Autodesk Fusion 360 part; units mm, degrees
note: some values were not read from the file. Chosen so that the rebuilt part matches the saved one: which bodies a step acts on; which face or edge a step refers to. Set by a fixed rule: which sketch regions a step uses.
(part 2 of 2)
extrude "Extrude3''" [suppressed] in component "Cube HalfSpace"
fillet "Fillet1''" [suppressed] in component "Cube HalfSpace"
extrude "Extrude4''" [suppressed] in component "Cube HalfSpace"
extrude "Extrude5''" [suppressed] in component "Cube HalfSpace"
extrude "Extrude6''" [suppressed] in component "Cube HalfSpace"
extrude "Extrude7''" [suppressed] in component "Cube HalfSpace"
fillet "Fillet2''" [suppressed] in component "Cube HalfSpace"
sketch "Sketch6 (3)" plane through (0, -18.4, 0) normal (0, -1, 0) x (1, 0, 0) in component "Cube HalfSpace"
  arc A0 (45.1, 20) -> (45.1, 10) centre (45.1, 15) ccw
  line L0 (45.1, 10) -> (50.15, 10)
  line L1 (50.15, 10) -> (50.15, 20)
  line L2 (50.15, 20) -> (45.1, 20)
  circle A1 centre (45.1, 15) radius 2.5
  circle A2 centre (45.1, 15) radius 5.1 construction
  dimension "d54_1" = 8.3333
  dimension "d63_1" = 16.8667
  constraint concentric A0 A1
  constraint concentric A0 A2
ref_plane "WorkPlane1" through (45.125, -20.9, 15) normal (0, -1, 0) x (1, 0, 0) in component "Cube HalfSpace"
sketch "Sketch7 (3)" plane through (35.7, -20.9, 16.5) normal (0, -1, 0) x (1, 0, 0) in component "Cube HalfSpace"
  point P0 (9.4, -1.5)
loft "Loft1''" [suppressed] in component "Cube HalfSpace"
sketch "Sketch8" plane through (0, -6.6, 0) normal (0, 1, 0) x (-1, 0, 0) in component "Cube HalfSpace"
  arc A0 (-45.1, 10) -> (-45.1, 20) centre (-45.1, 15) ccw
  line L0 (-45.1, 20) -> (-50.15, 20)
  line L1 (-50.15, 20) -> (-50.15, 10)
  line L2 (-50.15, 10) -> (-45.1, 10)
  circle A1 centre (-45.1, 15) radius 2.5
  circle A2 centre (-45.1, 15) radius 2.5
  dimension "d64_1" = 8.3333
  constraint concentric A1 A2
ref_plane "WorkPlane2" through (45.125, -4.1, 15) normal (0, 1, 0) x (-1, 0, 0) in component "Cube HalfSpace"
sketch "Sketch9" plane through (35.7, -4.1, 16.5) normal (0, 1, 0) x (1, 0, 0) in component "Cube HalfSpace"
  point P0 (9.4, 1.5)
loft "Loft2" [suppressed] in component "Cube HalfSpace"
sketch "Sketch10 (3)" plane through (0, -18.5, 0) normal (0, 1, 0) x (-1, 0, 0) in component "Cube HalfSpace"
  line L0 (-46.6, 20) -> (-50.1, 16.5)
  line L1 (-50.1, 16.5) -> (-50.1, 9.9)
  line L2 (-50.1, 9.9) -> (-40, 9.9)
  line L3 (-40, 9.9) -> (-40, 20)
  line L4 (-40, 20) -> (-46.6, 20)
  circle A0 centre (-45.1, 15) radius 2.5
  circle A1 centre (-45.1, 15) radius 2.6
  dimension "d57_1" = 0.1
ref_plane "WorkPlane3" through (36.3, -18.1, 16.2) normal (0, 1, 0) x (-1, 0, 0) in component "Cube HalfSpace"
sketch "Sketch11 (3)" plane through (35.4, -18.1, 16.3) normal (0, 1, 0) x (1, 0, 0) in component "Cube HalfSpace"
  point P0 (0.95, 0.05)
loft "Loft3''" [suppressed] in component "Cube HalfSpace"
ref_plane "WorkPlane4" through (30.1, -10, 20) normal (0, 1, 0) x (-1, 0, 0) in component "Cube HalfSpace"
mirror "Mirror1" [suppressed] in component "Cube HalfSpace"
ref_plane "WorkPlane5" through (10, -10, 20) normal (1, 0, 0) x (0, 1, 0) in component "Cube HalfSpace"
sketch "Sketch12 (3)" plane through (4.1, 0, 0) normal (-1, 0, 0) x (0, -1, 0) in component "Cube HalfSpace"
  arc A0 (3.75, 12.5) -> (3.75, 20) centre (3.75, 16.25) ccw
  line L0 (3.75, 20) -> (-0.05, 20)
  line L1 (-0.05, 20) -> (-0.05, 12.5)
  line L2 (-0.05, 12.5) -> (3.75, 12.5)
  circle A1 centre (3.75, 16.25) radius 2
  dimension "d66_1" = 8.3333
  constraint concentric A0 A1
ref_plane "WorkPlane6" through (2.1, -3.725, 16.25) normal (-1, 0, 0) x (0, -1, 0) in component "Cube HalfSpace"
sketch "Sketch13 (3)" plane through (2.1, -3.55, 16.25) normal (-1, 0, 0) x (0, 1, 0) in component "Cube HalfSpace"
  point P0 (-0.2, 0)
loft "Loft4''" [suppressed] in component "Cube HalfSpace"
sketch "Sketch14 (3)" plane through (4, 0, 0) normal (1, 0, 0) x (0, 1, 0) in component "Cube HalfSpace"
  line L0 (0, 16.5) -> (-3.5, 20)
  line L1 (-3.5, 20) -> (-7.6, 20)
  line L2 (-7.6, 20) -> (-7.6, 12.4)
  line L3 (-7.6, 12.4) -> (0, 12.4)
  line L4 (0, 12.4) -> (0, 16.5)
  circle A0 centre (-3.75, 16.25) radius 2
  circle A1 centre (-3.75, 16.25) radius 2.1
  dimension "d68_1" = 0.1
ref_plane "WorkPlane7" through (2.1, -3.8, 16.2) normal (1, 0, 0) x (0, 1, 0) in component "Cube HalfSpace"
sketch "Sketch15 (3)" plane through (2.1, -3.85, 16.05) normal (1, 0, 0) x (0, 1, 0) in component "Cube HalfSpace"
  point P0 (0.1, 0.2)
loft "Loft5''" [suppressed] in component "Cube HalfSpace"
mirror "Mirror2''" [suppressed] in component "Cube HalfSpace"
sketch "Sketch16 (3)" plane through (0, -4.1, 0) normal (0, 1, 0) x (-1, 0, 0) in component "Cube HalfSpace"
  arc A0 (-23.85, 7.5) -> (-23.85, 0) centre (-23.85, 3.75) ccw
  line L0 (-23.85, 0) -> (-16.25, 0)
  arc A1 (-16.25, 0) -> (-16.25, 7.5) centre (-16.25, 3.75) ccw
  line L1 (-16.25, 7.5) -> (-23.85, 7.5)
  circle A2 centre (-23.85, 3.75) radius 2
  circle A3 centre (-16.25, 3.75) radius 2
  dimension "d72_1" = 8.3333
  dimension "d73_1" = 8.3333
  constraint concentric A0 A2
  constraint concentric A1 A3
ref_plane "WorkPlane8" through (20.05, -2.1, 3.75) normal (0, 1, 0) x (-1, 0, 0) in component "Cube HalfSpace"
sketch "Sketch17 (3)" plane through (20.2, -2.1, 3.75) normal (0, 1, 0) x (1, 0, 0) in component "Cube HalfSpace"
  point P0 (3.65, 0)
  point P1 (-3.95, 0)
loft "Loft6''" [suppressed] in component "Cube HalfSpace"
loft "Loft7''" [suppressed] in component "Cube HalfSpace"
sketch "Sketch18 (3)" plane through (0, -4, 0) normal (0, -1, 0) x (1, 0, 0) in component "Cube HalfSpace"
  line L0 (16.5, 0) -> (20, 3.5)
  line L1 (20, 3.5) -> (20, 7.6)
  line L2 (20, 7.6) -> (12.4, 7.6)
  line L3 (12.4, 7.6) -> (12.4, 0)
  line L4 (12.4, 0) -> (16.5, 0)
  circle A0 centre (16.25, 3.75) radius 2
  circle A1 centre (16.25, 3.75) radius 2.1
  dimension "d75_1" = 0.1
ref_plane "WorkPlane9" through (16.2, -1.9, 3.8) normal (0, -1, 0) x (1, 0, 0) in component "Cube HalfSpace"
sketch "Sketch19 (3)" plane through (16.15, -1.9, 3.95) normal (0, -1, 0) x (1, 0, 0) in component "Cube HalfSpace"
  point P0 (0.1, -0.2)
loft "Loft8''" [suppressed] in component "Cube HalfSpace"
sketch "Sketch20 (3)" plane through (0, -4, 0) normal (0, -1, 0) x (1, 0, 0) in component "Cube HalfSpace"
  line L0 (20.1, 3.5) -> (23.6, 0)
  line L1 (23.6, 0) -> (27.7, 0)
  line L2 (27.7, 0) -> (27.7, 7.6)
  line L3 (27.7, 7.6) -> (20.1, 7.6)
  line L4 (20.1, 7.6) -> (20.1, 3.5)
  circle A0 centre (23.85, 3.75) radius 2
  circle A1 centre (23.85, 3.75) radius 2.1
  point P0 (23.85, 3.75)
  dimension "d77_1" = 0.1
ref_plane "WorkPlane10" through (23.9, -1.9, 3.8) normal (0, -1, 0) x (1, 0, 0) in component "Cube HalfSpace"
sketch "Sketch21 (3)" plane through (24.25, -1.9, 3.95) normal (0, -1, 0) x (1, 0, 0) in component "Cube HalfSpace"
  point P0 (-0.4, -0.2)
loft "Loft9''" [suppressed] in component "Cube HalfSpace"
mirror "Mirror3''" [suppressed] in component "Cube HalfSpace"
mirror "Mirror4''" [suppressed] in component "Cube HalfSpace"
combine "Combine2''" [suppressed] in component "Cube HalfSpace"
mirror "Mirror5''" [suppressed] in component "Cube HalfSpace"
combine "Combine3''" [suppressed] in component "Cube HalfSpace"
combine "Combine4''" [suppressed] in component "Cube HalfSpace"
sketch "Sketch1 (4)" plane through (0, 0, 0) normal (0, 0, 1) x (1, 0, 0) in component "Cube Hinge"
  line L0 (0, 0) -> (20, 0)
  line L1 (20, 0) -> (20, -20)
  line L2 (20, -20) -> (0, -20)
  line L3 (0, -20) -> (0, 0)
  line L4 (20.2, 0) -> (40.2, 0)
  line L5 (40.2, 0) -> (40.2, -20)
  line L6 (40.2, -20) -> (20.2, -20)
  line L7 (20.2, -20) -> (20.2, 0)
  dimension "d1_2" = 50
  dimension "d2_2" = 50
  dimension "d3_2" = 50
  dimension "d4_2" = 50
  dimension "d5_2" = 0.2
  constraint horizontal L0
  constraint vertical L1
  constraint horizontal L2
  constraint vertical L3
  constraint coincident L0.start L3.end
  constraint horizontal L4
  constraint vertical L5
  constraint horizontal L6
  constraint vertical L7
  constraint collinear L0 L4
  measures "d5_2" distance of L1 L7
extrude "Extrude1'''" [suppressed] in component "Cube Hinge"
sketch "Sketch2 (4)" plane through (0, 0, 0) normal (0, 0, -1) x (1, 0, 0) in component "Cube Hinge"
  line L0 (20, 20) -> (0, 20)
  line L1 (0, 20) -> (0, 0)
  line L2 (0, 0) -> (20, 0)
  line L3 (20, 0) -> (20, 20)
  line L4 (20, 4) -> (12.4, 4)
  line L5 (12.4, 4) -> (12.4, 16)
  line L6 (12.4, 16) -> (20, 16)
  line L7 (20, 16) -> (20, 4)
  line L8 (20.1, 4.2) -> (12.6, 4.2)
  line L9 (12.6, 4.2) -> (12.6, 15.8)
  line L10 (12.6, 15.8) -> (20.1, 15.8)
  line L11 (20.1, 15.8) -> (20.1, 4.2)
  line L12 (0, 10) -> (20, 10) construction
  dimension "d8_2" = 0.1
  dimension "d9_2" = 0.2
  dimension "d10_2" = 0.2
  dimension "d11_2" = 0.2
  dimension "d12_2" = 25
  dimension "d13_2" = 16.7667
  constraint horizontal L4
  constraint vertical L5
  constraint horizontal L6
  constraint vertical L7
  constraint coincident L3 L4.start
  constraint horizontal L8
  constraint vertical L9
  constraint horizontal L10
  constraint vertical L11
  constraint midpoint L1 L12.start
  constraint midpoint L3 L12.end
  constraint symmetric L4 L6 L12
  measures "d8_2" distance of L7 L11
  measures "d9_2" distance of L4 L8
  measures "d10_2" distance of L6 L10
  measures "d11_2" distance of L5 L9
sketch "Sketch3 (4)" plane through (0, 0, 0) normal (0, 0, -1) x (1, 0, 0) in component "Cube Hinge"
  line L0 (40.2, 20) -> (20.2, 20)
  line L1 (20.2, 20) -> (20.2, 0)
  line L2 (20.2, 0) -> (40.2, 0)
  line L3 (40.2, 0) -> (40.2, 20)
  line L4 (40.2, 10) -> (20.2, 10) construction
  line L5 (27.8, 4) -> (20.2, 4)
  line L6 (20.2, 4) -> (20.2, 16)
  line L7 (20.2, 16) -> (27.8, 16)
  line L8 (27.8, 16) -> (27.8, 4)
  line L9 (27.6, 4.2) -> (20.1, 4.2)
  line L10 (20.1, 4.2) -> (20.1, 15.8)
  line L11 (20.1, 15.8) -> (27.6, 15.8)
  line L12 (27.6, 15.8) -> (27.6, 4.2)
  dimension "d19_2" = 0.2
  dimension "d20_2" = 0.2
  dimension "d21_2" = 0.2
  dimension "d22_2" = 25
  dimension "d23_2" = 0.1
  dimension "d24_2" = 16.7667
  constraint midpoint L3 L4.start
  constraint midpoint L1 L4.end
  constraint horizontal L5
  constraint vertical L6
  constraint horizontal L7
  constraint vertical L8
  constraint coincident L1 L6.end
  constraint horizontal L9
  constraint vertical L10
  constraint horizontal L11
  constraint vertical L12
  constraint symmetric L4 L5 L7
  measures "d19_2" distance of L5 L9
  measures "d20_2" distance of L8 L12
  measures "d21_2" distance of L7 L11
  measures "d23_2" distance of L6 L10
sketch "Sketch4 (4)" plane through (0, 0, 20) normal (0, 0, 1) x (-1, 0, 0) in component "Cube Hinge"
  line L0 (0, 20) -> (-20, 20)
  line L1 (-20, 20) -> (-20, 0)
  line L2 (-20, 0) -> (0, 0)
  line L3 (0, 0) -> (0, 20)
  line L4 (-10, 20) -> (-10, 0) construction
  line L5 (-16, 7.6) -> (-4, 7.6)
  line L6 (-4, 7.6) -> (-4, 0)
  line L7 (-4, 0) -> (-16, 0)
  line L8 (-16, 0) -> (-16, 7.6)
  line L9 (-15.8, 7.4) -> (-4.2, 7.4)
  line L10 (-4.2, 7.4) -> (-4.2, -0.1)
  line L11 (-4.2, -0.1) -> (-15.8, -0.1)
  line L12 (-15.8, -0.1) -> (-15.8, 7.4)
  dimension "d25_2" = 0.1
  dimension "d26_2" = 0.2
  dimension "d27_2" = 0.2
  dimension "d28_2" = 25
  dimension "d29_2" = 0.2
  dimension "d30_2" = 16.7667
  constraint midpoint L0 L4.start
  constraint midpoint L2 L4.end
  constraint horizontal L5
  constraint vertical L6
  constraint horizontal L7
  constraint vertical L8
  constraint coincident L2 L6.end
  constraint horizontal L9
  constraint vertical L10
  constraint horizontal L11
  constraint vertical L12
  constraint symmetric L4 L6 L8
  measures "d25_2" distance of L7 L11
  measures "d26_2" distance of L8 L12
  measures "d27_2" distance of L6 L10
  measures "d29_2" distance of L5 L9
sketch "Sketch5 (4)" plane through (0, 0, 20) normal (0, 0, 1) x (-1, 0, 0) in component "Cube Hinge"
  line L0 (-20.2, 20) -> (-40.2, 20)
  line L1 (-40.2, 20) -> (-40.2, 0)
  line L2 (-40.2, 0) -> (-20.2, 0)
  line L3 (-20.2, 0) -> (-20.2, 20)
  line L4 (-40.2, 10) -> (-20.2, 10) construction
  line L5 (-40.2, 16) -> (-32.6, 16)
  line L6 (-32.6, 16) -> (-32.6, 4)
  line L7 (-32.6, 4) -> (-40.2, 4)
  line L8 (-40.2, 4) -> (-40.2, 16)
  line L9 (-40.3, 15.8) -> (-32.8, 15.8)
  line L10 (-32.8, 15.8) -> (-32.8, 4.2)
  line L11 (-32.8, 4.2) -> (-40.3, 4.2)
  line L12 (-40.3, 4.2) -> (-40.3, 15.8)
  dimension "d31_2" = 0.1
  dimension "d32_2" = 0.2
  dimension "d33_2" = 0.2
  dimension "d34_2" = 0.2
  dimension "d35_2" = 16.7667
  dimension "d36_2" = 25
  constraint midpoint L1 L4.start
  constraint midpoint L3 L4.end
  constraint horizontal L5
  constraint vertical L6
  constraint horizontal L7
  constraint vertical L8
  constraint coincident L1 L5.start
  constraint horizontal L9
  constraint vertical L10
  constraint horizontal L11
  constraint vertical L12
  constraint symmetric L4 L5 L7
  measures "d31_2" distance of L8 L12
  measures "d32_2" distance of L7 L11
  measures "d33_2" distance of L5 L9
  measures "d34_2" distance of L6 L10
chamfer "Chamfer1'''" [suppressed] in component "Cube Hinge"
extrude "Extrude2'''" [suppressed] in component "Cube Hinge"
extrude "Extrude3'''" [suppressed] in component "Cube Hinge"
fillet "Fillet1'''" [suppressed] in component "Cube Hinge"
sketch "Sketch16 (4)" plane through (0, -4.2, 0) normal (0, 1, 0) x (-1, 0, 0) in component "Cube Hinge"
  arc A0 (-23.85, 7.5) -> (-23.85, 0) centre (-23.85, 3.75) ccw
  line L0 (-23.85, 0) -> (-16.35, 0)
  arc A1 (-16.35, 0) -> (-16.35, 7.5) centre (-16.35, 3.75) ccw
  line L1 (-16.35, 7.5) -> (-23.85, 7.5)
  circle A2 centre (-23.85, 3.75) radius 2
  circle A3 centre (-16.35, 3.75) radius 2
  dimension "d72_2" = 8.3333
  dimension "d73_2" = 8.3333
  constraint concentric A0 A2
  constraint concentric A1 A3
ref_plane "WorkPlane8" through (20.1, -2.2, 3.75) normal (0, 1, 0) x (-1, 0, 0) in component "Cube Hinge"
sketch "Sketch17 (4)" plane through (20.2, -2.2, 3.75) normal (0, 1, 0) x (1, 0, 0) in component "Cube Hinge"
  point P0 (3.65, 0)
  point P1 (-3.85, 0)
loft "Loft6'''" [suppressed] in component "Cube Hinge"
loft "Loft7'''" [suppressed] in component "Cube Hinge"
sketch "Sketch18 (4)" plane through (0, -4, 0) normal (0, -1, 0) x (1, 0, 0) in component "Cube Hinge"
  line L0 (16.5, 0) -> (20, 3.5)
  line L1 (20, 3.5) -> (20, 7.7)
  line L2 (20, 7.7) -> (12.4, 7.7)
  line L3 (12.4, 7.7) -> (12.4, 0)
  line L4 (12.4, 0) -> (16.5, 0)
  circle A0 centre (16.35, 3.75) radius 2
  circle A1 centre (16.35, 3.75) radius 2.2
  dimension "d75_2" = 0.2
ref_plane "WorkPlane9" through (16.2, -1.9, 3.85) normal (0, -1, 0) x (1, 0, 0) in component "Cube Hinge"
sketch "Sketch19 (4)" plane through (16.15, -1.9, 3.95) normal (0, -1, 0) x (1, 0, 0) in component "Cube Hinge"
  point P0 (0.2, -0.2)
loft "Loft8'''" [suppressed] in component "Cube Hinge"
sketch "Sketch20 (4)" plane through (0, -4, 0) normal (0, -1, 0) x (1, 0, 0) in component "Cube Hinge"
  line L0 (20.2, 3.5) -> (23.7, 0)
  line L1 (23.7, 0) -> (27.8, 0)
  line L2 (27.8, 0) -> (27.8, 7.7)
  line L3 (27.8, 7.7) -> (20.2, 7.7)
  line L4 (20.2, 7.7) -> (20.2, 3.5)
  circle A0 centre (23.85, 3.75) radius 2
  circle A1 centre (23.85, 3.75) radius 2.2
  point P0 (23.85, 3.75)
  dimension "d77_2" = 0.2
ref_plane "WorkPlane10" through (24, -1.9, 3.85) normal (0, -1, 0) x (1, 0, 0) in component "Cube Hinge"
sketch "Sketch21 (4)" plane through (24.25, -1.9, 3.95) normal (0, -1, 0) x (1, 0, 0) in component "Cube Hinge"
  point P0 (-0.4, -0.2)
loft "Loft9'''" [suppressed] in component "Cube Hinge"
ref_plane "WorkPlane11" through (30.2, -10, 20) normal (0, 1, 0) x (-1, 0, 0) in component "Cube Hinge"
mirror "Mirror3'''" [suppressed] in component "Cube Hinge"
sketch "Sketch1 (5)" plane through (0, 0, 0) normal (0, 0, 1) x (1, 0, 0) in component "Cube Hinge HalfSpace"
  line L0 (0, 0) -> (20, 0)
  line L1 (20, 0) -> (20, -20)
  line L2 (20, -20) -> (0, -20)
  line L3 (0, -20) -> (0, 0)
  line L4 (20.1, 0) -> (40.1, 0)
  line L5 (40.1, 0) -> (40.1, -20)
  line L6 (40.1, -20) -> (20.1, -20)
  line L7 (20.1, -20) -> (20.1, 0)
  dimension "d1_2_1" = 50
  dimension "d2_2_1" = 50
  dimension "d3_2_1" = 50
  dimension "d4_2_1" = 50
  dimension "d5_2_1" = 0.1
  constraint horizontal L0
  constraint vertical L1
  constraint horizontal L2
  constraint vertical L3
  constraint coincident L0.start L3.end
  constraint horizontal L4
  constraint vertical L5
  constraint horizontal L6
  constraint vertical L7
  constraint collinear L0 L4
  measures "d5_2_1" distance of L1 L7
extrude "Extrude1''''" [suppressed] in component "Cube Hinge HalfSpace"
sketch "Sketch2 (5)" plane through (0, 0, 0) normal (0, 0, -1) x (1, 0, 0) in component "Cube Hinge HalfSpace"
  line L0 (20, 20) -> (0, 20)
  line L1 (0, 20) -> (0, 0)
  line L2 (0, 0) -> (20, 0)
  line L3 (20, 0) -> (20, 20)
  line L4 (20, 4) -> (12.4, 4)
  line L5 (12.4, 4) -> (12.4, 16)
  line L6 (12.4, 16) -> (20, 16)
  line L7 (20, 16) -> (20, 4)
  line L8 (20.05, 4.1) -> (12.5, 4.1)
  line L9 (12.5, 4.1) -> (12.5, 15.9)
  line L10 (12.5, 15.9) -> (20.05, 15.9)
  line L11 (20.05, 15.9) -> (20.05, 4.1)
  line L12 (0, 10) -> (20, 10) construction
  dimension "d8_2_1" = 0.05
  dimension "d9_2_1" = 0.1
  dimension "d10_2_1" = 0.1
  dimension "d11_2_1" = 0.1
  dimension "d12_2_1" = 25
  dimension "d13_2_1" = 16.7667
  constraint horizontal L4
  constraint vertical L5
  constraint horizontal L6
  constraint vertical L7
  constraint coincident L3 L4.start
  constraint horizontal L8
  constraint vertical L9
  constraint horizontal L10
  constraint vertical L11
  constraint midpoint L1 L12.start
  constraint midpoint L3 L12.end
  constraint symmetric L4 L6 L12
  measures "d8_2_1" distance of L7 L11
  measures "d9_2_1" distance of L4 L8
  measures "d10_2_1" distance of L6 L10
  measures "d11_2_1" distance of L5 L9
sketch "Sketch3 (5)" plane through (0, 0, 0) normal (0, 0, -1) x (1, 0, 0) in component "Cube Hinge HalfSpace"
  line L0 (40.1, 20) -> (20.1, 20)
  line L1 (20.1, 20) -> (20.1, 0)
  line L2 (20.1, 0) -> (40.1, 0)
  line L3 (40.1, 0) -> (40.1, 20)
  line L4 (40.1, 10) -> (20.1, 10) construction
  line L5 (27.7, 4) -> (20.1, 4)
  line L6 (20.1, 4) -> (20.1, 16)
  line L7 (20.1, 16) -> (27.7, 16)
  line L8 (27.7, 16) -> (27.7, 4)
  line L9 (27.6, 4.1) -> (20.05, 4.1)
  line L10 (20.05, 4.1) -> (20.05, 15.9)
  line L11 (20.05, 15.9) -> (27.6, 15.9)
  line L12 (27.6, 15.9) -> (27.6, 4.1)
  dimension "d19_2_1" = 0.1
  dimension "d20_2_1" = 0.1
  dimension "d21_2_1" = 0.1
  dimension "d22_2_1" = 25
  dimension "d23_2_1" = 0.05
  dimension "d24_2_1" = 16.7667
  constraint midpoint L3 L4.start
  constraint midpoint L1 L4.end
  constraint horizontal L5
  constraint vertical L6
  constraint horizontal L7
  constraint vertical L8
  constraint coincident L1 L6.end
  constraint horizontal L9
  constraint vertical L10
  constraint horizontal L11
  constraint vertical L12
  constraint symmetric L4 L5 L7
  measures "d19_2_1" distance of L5 L9
  measures "d20_2_1" distance of L8 L12
  measures "d21_2_1" distance of L7 L11
  measures "d23_2_1" distance of L6 L10
sketch "Sketch4 (5)" plane through (0, 0, 20) normal (0, 0, 1) x (-1, 0, 0) in component "Cube Hinge HalfSpace"
  line L0 (0, 20) -> (-20, 20)
  line L1 (-20, 20) -> (-20, 0)
  line L2 (-20, 0) -> (0, 0)
  line L3 (0, 0) -> (0, 20)
  line L4 (-10, 20) -> (-10, 0) construction
  line L5 (-16, 7.6) -> (-4, 7.6)
  line L6 (-4, 7.6) -> (-4, 0)
  line L7 (-4, 0) -> (-16, 0)
  line L8 (-16, 0) -> (-16, 7.6)
  line L9 (-15.8, 7.4) -> (-4.2, 7.4)
  line L10 (-4.2, 7.4) -> (-4.2, -0.1)
  line L11 (-4.2, -0.1) -> (-15.8, -0.1)
  line L12 (-15.8, -0.1) -> (-15.8, 7.4)
  dimension "d25_2_1" = 0.1
  dimension "d26_2_1" = 0.2
  dimension "d27_2_1" = 0.2
  dimension "d28_2_1" = 25
  dimension "d29_2_1" = 0.2
  dimension "d30_2_1" = 16.7667
  constraint midpoint L0 L4.start
  constraint midpoint L2 L4.end
  constraint horizontal L5
  constraint vertical L6
  constraint horizontal L7
  constraint vertical L8
  constraint coincident L2 L6.end
  constraint horizontal L9
  constraint vertical L10
  constraint horizontal L11
  constraint vertical L12
  constraint symmetric L4 L6 L8
  measures "d25_2_1" distance of L7 L11
  measures "d26_2_1" distance of L8 L12
  measures "d27_2_1" distance of L6 L10
  measures "d29_2_1" distance of L5 L9
sketch "Sketch5 (5)" plane through (0, 0, 20) normal (0, 0, 1) x (-1, 0, 0) in component "Cube Hinge HalfSpace"
  line L0 (-20.1, 20) -> (-40.1, 20)
  line L1 (-40.1, 20) -> (-40.1, 0)
  line L2 (-40.1, 0) -> (-20.1, 0)
  line L3 (-20.1, 0) -> (-20.1, 20)
  line L4 (-40.1, 10) -> (-20.1, 10) construction
  line L5 (-40.1, 16) -> (-32.5, 16)
  line L6 (-32.5, 16) -> (-32.5, 4)
  line L7 (-32.5, 4) -> (-40.1, 4)
  line L8 (-40.1, 4) -> (-40.1, 16)
  line L9 (-40.2, 15.8) -> (-32.7, 15.8)
  line L10 (-32.7, 15.8) -> (-32.7, 4.2)
  line L11 (-32.7, 4.2) -> (-40.2, 4.2)
  line L12 (-40.2, 4.2) -> (-40.2, 15.8)
  dimension "d31_2_1" = 0.1
  dimension "d32_2_1" = 0.2
  dimension "d33_2_1" = 0.2
  dimension "d34_2_1" = 0.2
  dimension "d35_2_1" = 16.7667
  dimension "d36_2_1" = 25
  constraint midpoint L1 L4.start
  constraint midpoint L3 L4.end
  constraint horizontal L5
  constraint vertical L6
  constraint horizontal L7
  constraint vertical L8
  constraint coincident L1 L5.start
  constraint horizontal L9
  constraint vertical L10
  constraint horizontal L11
  constraint vertical L12
  constraint symmetric L4 L5 L7
  measures "d31_2_1" distance of L8 L12
  measures "d32_2_1" distance of L7 L11
  measures "d33_2_1" distance of L5 L9
  measures "d34_2_1" distance of L6 L10
chamfer "Chamfer1''''" [suppressed] in component "Cube Hinge HalfSpace"
extrude "Extrude2''''" [suppressed] in component "Cube Hinge HalfSpace"
extrude "Extrude3''''" [suppressed] in component "Cube Hinge HalfSpace"
fillet "Fillet1''''" [suppressed] in component "Cube Hinge HalfSpace"
sketch "Sketch16 (5)" plane through (0, -4.1, 0) normal (0, 1, 0) x (-1, 0, 0) in component "Cube Hinge HalfSpace"
  arc A0 (-23.85, 7.5) -> (-23.85, 0) centre (-23.85, 3.75) ccw
  line L0 (-23.85, 0) -> (-16.25, 0)
  arc A1 (-16.25, 0) -> (-16.25, 7.5) centre (-16.25, 3.75) ccw
  line L1 (-16.25, 7.5) -> (-23.85, 7.5)
  circle A2 centre (-23.85, 3.75) radius 2
  circle A3 centre (-16.25, 3.75) radius 2
  dimension "d72_2_1" = 8.3333
  dimension "d73_2_1" = 8.3333
  constraint concentric A0 A2
  constraint concentric A1 A3
ref_plane "WorkPlane8" through (20.05, -2.1, 3.75) normal (0, 1, 0) x (-1, 0, 0) in component "Cube Hinge HalfSpace"
sketch "Sketch17 (5)" plane through (20.2, -2.1, 3.75) normal (0, 1, 0) x (1, 0, 0) in component "Cube Hinge HalfSpace"
  point P0 (3.65, 0)
  point P1 (-3.95, 0)
loft "Loft6''''" [suppressed] in component "Cube Hinge HalfSpace"
loft "Loft7''''" [suppressed] in component "Cube Hinge HalfSpace"
sketch "Sketch18 (5)" plane through (0, -4, 0) normal (0, -1, 0) x (1, 0, 0) in component "Cube Hinge HalfSpace"
  line L0 (16.5, 0) -> (20, 3.5)
  line L1 (20, 3.5) -> (20, 7.6)
  line L2 (20, 7.6) -> (12.4, 7.6)
  line L3 (12.4, 7.6) -> (12.4, 0)
  line L4 (12.4, 0) -> (16.5, 0)
  circle A0 centre (16.25, 3.75) radius 2
  circle A1 centre (16.25, 3.75) radius 2.2
  dimension "d75_2_1" = 0.2
ref_plane "WorkPlane9" through (16.2, -1.9, 3.8) normal (0, -1, 0) x (1, 0, 0) in component "Cube Hinge HalfSpace"
sketch "Sketch19 (5)" plane through (16.15, -1.9, 3.95) normal (0, -1, 0) x (1, 0, 0) in component "Cube Hinge HalfSpace"
  point P0 (0.1, -0.2)
loft "Loft8''''" [suppressed] in component "Cube Hinge HalfSpace"
sketch "Sketch20 (5)" plane through (0, -4, 0) normal (0, -1, 0) x (1, 0, 0) in component "Cube Hinge HalfSpace"
  line L0 (20.1, 3.5) -> (23.6, 0)
  line L1 (23.6, 0) -> (27.7, 0)
  line L2 (27.7, 0) -> (27.7, 7.6)
  line L3 (27.7, 7.6) -> (20.1, 7.6)
  line L4 (20.1, 7.6) -> (20.1, 3.5)
  circle A0 centre (23.85, 3.75) radius 2
  circle A1 centre (23.85, 3.75) radius 2.2
  point P0 (23.85, 3.75)
  dimension "d77_2_1" = 0.2
ref_plane "WorkPlane10" through (23.9, -1.9, 3.8) normal (0, -1, 0) x (1, 0, 0) in component "Cube Hinge HalfSpace"
sketch "Sketch21 (5)" plane through (24.25, -1.9, 3.95) normal (0, -1, 0) x (1, 0, 0) in component "Cube Hinge HalfSpace"
  point P0 (-0.4, -0.2)
loft "Loft9''''" [suppressed] in component "Cube Hinge HalfSpace"
ref_plane "WorkPlane11" through (30.1, -10, 20) normal (0, 1, 0) x (-1, 0, 0) in component "Cube Hinge HalfSpace"
mirror "Mirror3''''" [suppressed] in component "Cube Hinge HalfSpace"
component "Cube" placed x (1, 0, 0) y (0, 1, 0) z (0, 0, 1) at (0, 0, 0)
component "Holey Cube" placed x (1, 0, 0) y (0, 1, 0) z (0, 0, 1) at (0, 0, 0)
equation "d1 = cube_edge"
equation "d2 = cube_edge"
equation "d3 = cube_edge"
equation "d4 = cube_edge"
equation "d5 = clearance"
equation "d6 = cube_edge"
equation "d8 = clearance / 2"
equation "d9 = clearance"
equation "d10 = clearance"
equation "d11 = clearance"
equation "d12 = hinge_width"
equation "d13 = half_hinge_length"
equation "cube_edge = 50 mm"
equation "half_hinge_length = hinge_thickness + clearance / 2"
equation "hinge_width = ( cube_edge / 2 mm ) * 1 mm"
equation "hinge_thickness = ( cube_edge / 3 mm ) * 1 mm"
equation "clearance = 0.2 mm"
equation "d19 = clearance"
equation "d20 = clearance"
equation "d21 = clearance"
equation "d22 = hinge_width"
equation "d23 = clearance / 2"
equation "d24 = half_hinge_length"
equation "d25 = clearance / 2"
equation "d26 = clearance"
equation "d27 = clearance"
equation "d28 = hinge_width"
equation "d29 = clearance"
equation "d30 = half_hinge_length"
equation "d37 = chamfer"
equation "d38 = -hinge_thickness - clearance"
equation "d40 = -hinge_thickness"
equation "d43 = hinge_thickness / 2"
equation "d44 = -hinge_thickness - clearance"
equation "d46 = -hinge_thickness - clearance"
equation "d48 = -hinge_thickness"
equation "d50 = -hinge_thickness"
equation "d53 = hinge_thickness / 2"
equation "d55 = -hinge_pin_diameter / 2 - clearance / 2"
equation "d58 = hinge_pin_diameter / 2"
equation "hinge_pin_diameter = ( hinge_thickness * 1 / 2 mm ) * 1 mm"
equation "d66 = hinge_pin_diameter"
equation "d67 = hinge_pin_diameter / 2"
equation "d69 = -hinge_pin_diameter / 2 + clearance / 2"
equation "d72 = hinge_pin_diameter"
equation "d73 = hinge_pin_diameter"
equation "d74 = hinge_pin_diameter / 2"
equation "d75 = clearance * 1.5"
equation "d76 = -hinge_pin_diameter / 2 - clearance / 2"
equation "d77 = clearance * 1.5"
equation "d78 = -hinge_pin_diameter / 2 - clearance / 2"
equation "d1_1 = cube_edge"
equation "d2_1 = cube_edge"
equation "d3_1 = cube_edge"
equation "d4_1 = cube_edge"
equation "d5_1 = clearance / 2"
equation "d8_1 = clearance / 4"
equation "d9_1 = clearance / 2"
equation "d10_1 = clearance / 2"
equation "d11_1 = clearance / 2"
equation "d12_1 = hinge_width"
equation "d13_1 = half_hinge_length"
equation "d19_1 = clearance / 2"
equation "d20_1 = clearance / 2"
equation "d21_1 = clearance / 2"
equation "d22_1 = hinge_width"
equation "d23_1 = clearance / 4"
equation "d24_1 = half_hinge_length"
equation "d25_1 = clearance / 4"
equation "d26_1 = clearance / 2"
equation "d27_1 = clearance / 2"
equation "d28_1 = hinge_width"
equation "d29_1 = clearance / 2"
equation "d30_1 = half_hinge_length"
equation "d31_1 = clearance / 4"
equation "d32_1 = clearance / 2"
equation "d33_1 = clearance / 2"
equation "d34_1 = clearance / 2"
equation "d35_1 = half_hinge_length"
equation "d36_1 = hinge_width"
equation "d38_1 = -hinge_thickness - clearance / 2"
equation "d40_1 = -hinge_thickness"
equation "d43_1 = hinge_thickness / 2"
equation "d44_1 = -hinge_thickness - clearance / 2"
equation "d46_1 = -hinge_thickness - clearance / 2"
equation "d48_1 = -hinge_thickness"
equation "d50_1 = -hinge_thickness"
equation "d53_1 = hinge_thickness / 2"
equation "d54_1 = hinge_pin_diameter"
equation "d55_1 = hinge_pin_diameter / 2"
equation "d56_1 = hinge_pin_diameter / 2"
equation "d57_1 = clearance / 2"
equation "d58_1 = -hinge_pin_diameter / 2 - clearance / 2"
equation "d63_1 = half_hinge_length * 2 - hinge_thickness"
equation "d64_1 = hinge_pin_diameter"
equation "d66_1 = hinge_pin_diameter"
equation "d67_1 = hinge_pin_diameter / 2"
equation "d68_1 = clearance / 2"
equation "d69_1 = -hinge_pin_diameter / 2 + clearance / 2"
equation "d72_1 = hinge_pin_diameter"
equation "d73_1 = hinge_pin_diameter"
equation "d74_1 = hinge_pin_diameter / 2"
equation "d75_1 = clearance / 2"
equation "d76_1 = -hinge_pin_diameter / 2 - clearance / 2"
equation "d77_1 = clearance / 2"
equation "d78_1 = -hinge_pin_diameter / 2 - clearance / 2"
equation "d1_2 = cube_edge"
equation "d2_2 = cube_edge"
equation "d3_2 = cube_edge"
equation "d4_2 = cube_edge"
equation "d5_2 = clearance"
equation "d8_2 = clearance / 2"
equation "d9_2 = clearance"
equation "d10_2 = clearance"
equation "d11_2 = clearance"
equation "d12_2 = hinge_width"
equation "d13_2 = half_hinge_length"
equation "d19_2 = clearance"
equation "d20_2 = clearance"
equation "d21_2 = clearance"
equation "d22_2 = hinge_width"
equation "d23_2 = clearance / 2"
equation "d24_2 = half_hinge_length"
equation "d25_2 = clearance / 2"
equation "d26_2 = clearance"
equation "d27_2 = clearance"
equation "d28_2 = hinge_width"
equation "d29_2 = clearance"
equation "d30_2 = half_hinge_length"
equation "d31_2 = clearance / 2"
equation "d32_2 = clearance"
equation "d33_2 = clearance"
equation "d34_2 = clearance"
equation "d35_2 = half_hinge_length"
equation "d36_2 = hinge_width"
equation "d38_2 = -hinge_thickness - clearance"
equation "d40_2 = -hinge_thickness"
equation "d43_2 = hinge_thickness / 2"
equation "d72_2 = hinge_pin_diameter"
equation "d73_2 = hinge_pin_diameter"
equation "d74_2 = hinge_pin_diameter / 2"
equation "d75_2 = clearance"
equation "d76_2 = -hinge_pin_diameter / 2 - clearance / 2"
equation "d77_2 = clearance"
equation "d78_2 = -hinge_pin_diameter / 2 - clearance / 2"
equation "d1_2_1 = cube_edge"
equation "d2_2_1 = cube_edge"
equation "d3_2_1 = cube_edge"
equation "d4_2_1 = cube_edge"
equation "d5_2_1 = clearance / 2"
equation "d8_2_1 = clearance / 4"
equation "d9_2_1 = clearance / 2"
equation "d10_2_1 = clearance / 2"
equation "d11_2_1 = clearance / 2"
equation "d12_2_1 = hinge_width"
equation "d13_2_1 = half_hinge_length"
equation "d19_2_1 = clearance / 2"
equation "d20_2_1 = clearance / 2"
equation "d21_2_1 = clearance / 2"
equation "d22_2_1 = hinge_width"
equation "d23_2_1 = clearance / 4"
equation "d24_2_1 = half_hinge_length"
equation "d25_2_1 = clearance / 2"
equation "d26_2_1 = clearance"
equation "d27_2_1 = clearance"
equation "d28_2_1 = hinge_width"
equation "d29_2_1 = clearance"
equation "d30_2_1 = half_hinge_length"
equation "d31_2_1 = clearance / 2"
equation "d32_2_1 = clearance"
equation "d33_2_1 = clearance"
equation "d34_2_1 = clearance"
equation "d35_2_1 = half_hinge_length"
equation "d36_2_1 = hinge_width"
equation "d38_2_1 = -hinge_thickness - clearance / 2"
equation "d40_2_1 = -hinge_thickness"
equation "d43_2_1 = hinge_thickness / 2"
equation "d72_2_1 = hinge_pin_diameter"
equation "d73_2_1 = hinge_pin_diameter"
equation "d74_2_1 = hinge_pin_diameter / 2"
equation "d75_2_1 = clearance"
equation "d76_2_1 = -hinge_pin_diameter / 2 - clearance / 2"
equation "d77_2_1 = clearance"
equation "d78_2_1 = -hinge_pin_diameter / 2 - clearance / 2"
equation "d87 = half_hinge_length"
equation "d88 = clearance"
equation "d89 = clearance"
equation "d90 = clearance"
equation "d91 = hinge_width"
equation "d92 = clearance / 2"
equation "d94 = hinge_thickness / 2"
equation "d95 = hinge_pin_diameter"
equation "chamfer = hinge_thickness / 2"
equation "d101 = clearance"
equation "d102 = clearance * 1.5"
equation "d103 = hinge_pin_diameter"
equation "d104 = hinge_pin_diameter"
equation "d105 = hinge_pin_diameter / 2"
equation "d106 = hinge_pin_diameter + clearance * 1.5"
equation "d107 = -hinge_pin_diameter / 2 - clearance / 2"
equation "d108 = hinge_pin_diameter + clearance * 1.5"
equation "inside_chamfer = chamfer / 8"
equation "d1_4 = cube_edge"
equation "d2_4 = cube_edge"
equation "d3_4 = cube_edge"
equation "d4_4 = cube_edge"
equation "d5_4 = clearance"
equation "d6_4 = cube_edge"
equation "d8_4 = clearance / 2"
equation "d9_4 = clearance"
equation "d10_4 = clearance"
equation "d11_4 = clearance"
equation "d12_4 = hinge_width"
equation "d13_4 = half_hinge_length"
equation "d19_4 = clearance"
equation "d20_4 = clearance"
equation "d21_4 = clearance"
equation "d22_4 = hinge_width"
equation "d23_4 = clearance / 2"
equation "d24_4 = half_hinge_length"
equation "d25_4 = clearance / 2"
equation "d26_4 = clearance"
equation "d27_4 = clearance"
equation "d28_4 = hinge_width"
equation "d29_4 = clearance"
equation "d30_4 = half_hinge_length"
equation "d37_4 = chamfer"
equation "d38_4 = -hinge_thickness - clearance"
equation "d40_4 = -hinge_thickness"
equation "d43_4 = hinge_thickness / 2"
equation "d44_3 = -hinge_thickness - clearance"
equation "d46_3 = -hinge_thickness - clearance"
equation "d48_3 = -hinge_thickness"
equation "d50_3 = -hinge_thickness"
equation "d53_3 = hinge_thickness / 2"
equation "d55_2 = -hinge_pin_diameter / 2 - clearance / 2"
equation "d58_2 = hinge_pin_diameter / 2"
equation "d66_3 = hinge_pin_diameter"
equation "d67_3 = hinge_pin_diameter / 2"
equation "d69_2 = -hinge_pin_diameter / 2 + clearance / 2"
equation "d72_4 = hinge_pin_diameter"
equation "d73_4 = hinge_pin_diameter"
equation "d74_3 = hinge_pin_diameter / 2"
equation "d75_3 = clearance * 1.5"
equation "d76_3 = -hinge_pin_diameter / 2 - clearance / 2"
equation "d77_3 = clearance * 1.5"
equation "d78_3 = -hinge_pin_diameter / 2 - clearance / 2"
equation "d87_2 = half_hinge_length"
equation "d88_2 = clearance"
equation "d89_2 = clearance"
equation "d90_2 = clearance"
equation "d91_2 = hinge_width"
equation "d92_2 = clearance / 2"
equation "d94_2 = hinge_thickness / 2"
equation "d95_2 = hinge_pin_diameter"
equation "d101_1 = clearance"
equation "d102_2 = clearance * 1.5"
equation "d103_1 = hinge_pin_diameter"
equation "d104_1 = hinge_pin_diameter"
equation "d105_1 = hinge_pin_diameter / 2"
equation "d106_1 = hinge_pin_diameter + clearance * 1.5"
equation "d107_1 = -hinge_pin_diameter / 2 - clearance / 2"
equation "d108_2 = hinge_pin_diameter + clearance * 1.5"
equation "d154 = hinge_width"
equation "d155 = hinge_width"
equation "d158 = hinge_width"
equation "d159 = hinge_width"
equation "d162 = hinge_width"
equation "d163 = hinge_width"
equation "d166 = hinge_width"
equation "d167 = hinge_width"
equation "d174 = inside_chamfer"
equation "d175 = hinge_width"
equation "d176 = hinge_width"
